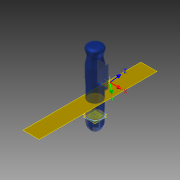
# Autodesk Inventor part: Handle_2
Saved by Autodesk Inventor 2011 SP2 (Build 150309200, 309)
## iProperties
Created: 2012-02-26
Part Number: Handle_2
Document SubType Name: Modeling
Designer: sungwook
Density: 1 g/cm^3
Author: sungwook
Autodesk Inventor part; units mm, degrees
note: some values were not read from the file. Chosen so that the rebuilt part matches the saved one: direction of "Hole2".
(part 1 of 20)
ref_plane "YZ Plane" through (0, 0, 0) normal (1, 0, 0) x (0, 1, 0)
sketch "Handle_0" plane through (0, 0, 0) normal (0, 0, 1) x (1, 0, 0)
  spline S0 degree 3 poles (-10017.42764, -10030.297385) (-10017.013951, -10030.15636) (-10016.17375, -10029.86994) (-10014.867675, -10029.493529) (-10013.491481, -10029.172596) (-10012.078899, -10028.93448) (-10010.677748, -10028.78461) (-10009.329448, -10028.709162) (-10008.026956, -10028.683902) (-10007.172289, -10028.683862) (-10006.749998, -10028.683842) knots 0 0 0 0 0.13110718 0.26627767 0.40758133 0.55482273 0.69573025 0.83010398 0.95981582 1.08650249 1.08650249 1.08650249 1.08650249
  spline S1 degree 3 poles (-10021.732129, -10032.297385) (-10021.73234, -10032.297385) (-10021.733186, -10032.297385) (-10021.73509, -10032.297385) (-10021.738258, -10032.297385) (-10021.742688, -10032.297385) (-10021.748373, -10032.297385) (-10021.755307, -10032.297385) (-10021.763486, -10032.297385) (-10021.772904, -10032.297385) (-10021.783555, -10032.297385) (-10021.795433, -10032.297385) (-10021.808523, -10032.297385) (-10021.822807, -10032.297385) (-10021.838268, -10032.297385) (-10021.854892, -10032.297385) (-10021.872666, -10032.297385) (-10021.884898, -10032.297385) (-10021.891203, -10032.297385) knots 0 0 0 0 0.00398745 0.01595749 0.03589091 0.06374884 0.09949715 0.14310174 0.1945285 0.2537433 0.32071204 0.39540061 0.47774624 0.56757484 0.66479437 0.76932497 0.8810868 1 1 1 1
  spline S2 degree 3 poles (-10021.891203, -10032.297385) (-10021.507581, -10032.143895) (-10020.74627, -10031.83929) (-10019.261429, -10031.164287) (-10018.160679, -10030.64392) (-10017.42764, -10030.297385) knots 0 0 0 0 0.25334256 0.50276707 1 1 1 1
  spline S3 degree 3 poles (-10017.79088, -10013.983385) (-10017.364369, -10014.133003) (-10016.497172, -10014.437213) (-10015.148667, -10014.843297) (-10013.724339, -10015.192835) (-10012.260529, -10015.454201) (-10010.808862, -10015.619234) (-10009.414249, -10015.702378) (-10008.068673, -10015.730197) (-10007.18611, -10015.730238) (-10006.749998, -10015.730259) knots 0 0 0 0 0.13558682 0.27568002 0.42231514 0.57532331 0.7214304 0.86036495 0.99429907 1.12513191 1.12513191 1.12513191 1.12513191
  line L0 (-10022.303899, -10015.983385) -> (-10006.749998, -10015.983385)
  line L1 (-10006.749998, -10015.730259) -> (-10006.749998, -10015.983385)
  line L2 (-10006.749998, -10015.983385) -> (-10006.749998, -10017.983385)
  spline S4 degree 3 poles (-10006.749998, -10017.983385) (-10007.632309, -10017.983385) (-10008.976773, -10017.983385) (-10010.804987, -10017.983385) (-10012.253003, -10017.983385) (-10013.713888, -10017.983385) (-10015.138402, -10017.983385) (-10016.48847, -10017.983385) (-10017.363516, -10017.983385) (-10017.791183, -10017.983385) knots 0 0 0 0 0.26469338 0.4033392 0.54846434 0.69909791 0.84160494 0.97581833 1.10411856 1.10411856 1.10411856 1.10411856
  spline S5 degree 3 poles (-10017.791183, -10017.983385) (-10018.527422, -10017.630624) (-10019.634362, -10017.100245) (-10020.947309, -10016.51954) (-10021.715083, -10016.204989) (-10022.106855, -10016.057543) (-10022.303899, -10015.983385) knots 0 0 0 0 0.49596798 0.74569065 0.8720938 1 1 1 1
  spline S6 degree 3 poles (-10022.303899, -10015.983385) (-10022.278889, -10015.901813) (-10022.229009, -10015.739129) (-10022.178389, -10015.489096) (-10022.146804, -10015.236972) (-10022.136391, -10014.983317) (-10022.146773, -10014.729742) (-10022.178339, -10014.477516) (-10022.22892, -10014.227552) (-10022.278782, -10014.064856) (-10022.303752, -10013.983385) knots 0 0 0 0 0.12572609 0.25074567 0.37552827 0.50000542 0.62458391 0.74924522 0.87443269 1 1 1 1
  spline S7 degree 3 poles (-10022.303752, -10013.983385) (-10021.914411, -10013.983385) (-10021.148705, -10013.983385) (-10019.644415, -10013.983385) (-10018.529465, -10013.983385) (-10017.79088, -10013.983385) knots 0 0 0 0 0.25882001 0.5090148 1 1 1 1
  line L3 (-10033.249998, -10030.297385) -> (-10017.42764, -10030.297385)
  line L4 (-10033.249998, -10030.297385) -> (-10033.249998, -10028.297385)
  line L5 (-10033.249998, -10028.297385) -> (-10006.749998, -10028.297385)
  line L6 (-10033.249998, -10032.297385) -> (-10021.891203, -10032.297385)
  line L7 (-10033.249998, -10032.297385) -> (-10033.249998, -10030.297385)
  line L8 (-10033.249998, -10017.983385) -> (-10017.791183, -10017.983385)
  line L9 (-10033.249998, -10017.983385) -> (-10033.249998, -10015.983385)
  line L10 (-10033.249998, -10015.983385) -> (-10022.303899, -10015.983385)
  line L11 (-10033.249998, -10015.983385) -> (-10033.249998, -10013.983385)
  line L12 (-10033.249998, -10013.983385) -> (-10022.303752, -10013.983385)
  line L13 (-10033.249998, -10018.729385) -> (-10006.749998, -10018.729385)
  line L14 (-10033.249998, -10018.729385) -> (-10033.249998, -10017.983385)
  line L15 (-10033.249998, -10016.729385) -> (-10006.749998, -10016.729385)
  line L16 (-10033.249998, -10014.729385) -> (-10017.28307, -10014.729385)
  spline S8 degree 3 poles (-10006.749998, -10016.350628) (-10007.166577, -10016.350609) (-10008.009501, -10016.35057) (-10009.293989, -10016.325181) (-10010.623578, -10016.249325) (-10012.005692, -10016.098622) (-10013.399659, -10015.859202) (-10014.758004, -10015.536726) (-10016.046768, -10015.158729) (-10016.875274, -10014.871005) (-10017.28307, -10014.729385) knots 0 0 0 0 0.12497306 0.25287553 0.38537145 0.52436553 0.66974205 0.80937847 0.9429718 1.07246485 1.07246485 1.07246485 1.07246485
  spline S9 degree 3 poles (-10022.047249, -10014.729385) (-10022.04174, -10014.815541) (-10022.030727, -10014.987752) (-10022.041635, -10015.246826) (-10022.072516, -10015.50434) (-10022.12485, -10015.759276) (-10022.197222, -10016.010445) (-10022.289119, -10016.256609) (-10022.398025, -10016.497644) (-10022.48411, -10016.651957) (-10022.527304, -10016.729385) knots 0 0 0 0 0.12386032 0.2475762 0.37158497 0.495852 0.6207493 0.74643209 0.87276965 1 1 1 1
  spline S10 degree 3 poles (-10022.527304, -10016.729385) (-10022.341346, -10016.801452) (-10021.971207, -10016.944898) (-10021.245451, -10017.252698) (-10020.356992, -10017.662141) (-10019.309622, -10018.185828) (-10018.619278, -10018.548029) (-10018.273621, -10018.729385) knots 0 0 0 0 0.12719878 0.25318248 0.50275428 0.75102731 1 1 1 1
  line L17 (-10035.749998, -10008.803385) -> (-10035.749998, -10032.803385)
  line L18 (-10149.710906, -10011.319385) -> (-10149.710906, -10030.287385)
  line L19 (-10149.325539, -10010.832703) -> (-10149.325539, -10030.774067)
  spline S11 degree 3 poles (-10130.726906, -10031.787385) (-10130.926034, -10031.641629) (-10131.327631, -10031.347673) (-10132.100995, -10030.700181) (-10132.860268, -10030.021094) (-10133.656819, -10029.374911) (-10134.185656, -10029.005591) (-10134.632315, -10028.744292) (-10134.982155, -10028.568235) (-10135.346656, -10028.411869) (-10135.59944, -10028.329114) (-10135.726906, -10028.287385) knots 0 0 0 0 0.07401284 0.14926686 0.30244691 0.37959616 0.45685507 0.49566205 0.53474567 0.5742877 0.61450742 0.61450742 0.61450742 0.61450742
  spline S12 degree 3 poles (-10130.726906, -10009.819385) (-10130.926034, -10009.965141) (-10131.327631, -10010.259097) (-10132.100995, -10010.906589) (-10132.860268, -10011.585676) (-10133.656819, -10012.231858) (-10134.185656, -10012.601179) (-10134.632315, -10012.862478) (-10134.982155, -10013.038535) (-10135.346656, -10013.194901) (-10135.59944, -10013.277656) (-10135.726906, -10013.319385) knots 0 0 0 0 0.07401284 0.14926686 0.30244691 0.37959616 0.45685507 0.49566205 0.53474567 0.5742877 0.61450742 0.61450742 0.61450742 0.61450742
  spline S13 degree 3 poles (-10125.726906, -10033.303385) (-10125.949716, -10033.300239) (-10126.395062, -10033.29395) (-10127.059625, -10033.234489) (-10127.71554, -10033.128934) (-10128.357478, -10032.969394) (-10128.981847, -10032.754825) (-10129.585717, -10032.484089) (-10130.170679, -10032.163086) (-10130.540701, -10031.913156) (-10130.726906, -10031.787385) knots 0 0 0 0 0.06683217 0.13358148 0.19996019 0.26595386 0.33177154 0.39774949 0.46426825 0.53165054 0.53165054 0.53165054 0.53165054
  spline S14 degree 3 poles (-10125.726906, -10008.303385) (-10125.949716, -10008.306531) (-10126.395062, -10008.312819) (-10127.059625, -10008.37228) (-10127.71554, -10008.477836) (-10128.357478, -10008.637376) (-10128.981847, -10008.851945) (-10129.585717, -10009.12268) (-10130.170679, -10009.443684) (-10130.540701, -10009.693614) (-10130.726906, -10009.819385) knots 0 0 0 0 0.06683217 0.13358148 0.19996019 0.26595386 0.33177154 0.39774949 0.46426825 0.53165054 0.53165054 0.53165054 0.53165054
  arc A0 (-10149.325539, -10010.832703) -> (-10149.710906, -10011.319385) centre (-10149.210906, -10011.319385) ccw
  arc A1 (-10149.710906, -10030.287385) -> (-10149.325539, -10030.774067) centre (-10149.210906, -10030.287385) ccw
  spline S15 degree 3 poles (-10135.726906, -10028.287385) (-10135.927757, -10028.233252) (-10136.338929, -10028.122433) (-10136.990756, -10028.038079) (-10137.683253, -10028.010641) (-10138.418457, -10028.048208) (-10139.194997, -10028.144543) (-10140.011682, -10028.296223) (-10140.865557, -10028.499181) (-10142.071793, -10028.832792) (-10143.629971, -10029.328885) (-10145.526237, -10029.953098) (-10147.128782, -10030.412477) (-10148.397883, -10030.680686) (-10149.021234, -10030.743434) (-10149.325539, -10030.774067) knots 0 0 0 0 0.06234657 0.1276327 0.1966407 0.27004939 0.34820305 0.43123424 0.51911498 0.61142292 0.80662861 1.00959387 1.21035176 1.30648489 1.39817641 1.39817641 1.39817641 1.39817641
  spline S16 degree 3 poles (-10135.726906, -10013.319385) (-10135.927757, -10013.373518) (-10136.338929, -10013.484337) (-10136.990756, -10013.56869) (-10137.683253, -10013.596129) (-10138.418457, -10013.558561) (-10139.194997, -10013.462227) (-10140.011682, -10013.310547) (-10140.865557, -10013.107589) (-10142.071793, -10012.773978) (-10143.629971, -10012.277884) (-10145.526237, -10011.653672) (-10147.128782, -10011.194293) (-10148.397883, -10010.926084) (-10149.021234, -10010.863335) (-10149.325539, -10010.832703) knots 0 0 0 0 0.06234657 0.1276327 0.1966407 0.27004939 0.34820305 0.43123424 0.51911498 0.61142292 0.80662861 1.00959387 1.21035176 1.30648489 1.39817641 1.39817641 1.39817641 1.39817641
  line L20 (-10150.726906, -10009.803385) -> (-10150.726906, -10031.803385)
  spline S17 degree 3 poles (-10135.726906, -10029.303385) (-10135.510838, -10029.403925) (-10135.07407, -10029.607162) (-10134.444184, -10029.982096) (-10133.812917, -10030.390211) (-10133.179963, -10030.831085) (-10132.5504, -10031.300817) (-10131.733284, -10031.962031) (-10131.128514, -10032.467631) (-10130.726906, -10032.803385) knots 0 0 0 0 0.07145122 0.1444341 0.21963753 0.29697342 0.37578786 0.45523025 0.61227239 0.61227239 0.61227239 0.61227239
  spline S18 degree 3 poles (-10135.726906, -10012.303385) (-10135.510838, -10012.202844) (-10135.07407, -10011.999608) (-10134.444184, -10011.624673) (-10133.812917, -10011.216558) (-10133.179963, -10010.775684) (-10132.5504, -10010.305952) (-10131.733284, -10009.644738) (-10131.128514, -10009.139138) (-10130.726906, -10008.803385) knots 0 0 0 0 0.07145122 0.1444341 0.21963753 0.29697342 0.37578786 0.45523025 0.61227239 0.61227239 0.61227239 0.61227239
  spline S19 degree 3 poles (-10130.726906, -10032.803385) (-10130.542266, -10032.946932) (-10130.26739, -10033.160633) (-10129.883991, -10033.41627) (-10129.594046, -10033.590111) (-10129.298537, -10033.745569) (-10128.997284, -10033.882043) (-10128.689809, -10033.998389) (-10128.376285, -10034.094702) (-10128.057096, -10034.171953) (-10127.623115, -10034.250453) (-10127.069205, -10034.306035) (-10126.399156, -10034.322456) (-10125.950896, -10034.320408) (-10125.726906, -10034.319385) knots 0 0 0 0 0.07013118 0.1044054 0.13817293 0.17150982 0.2045203 0.23732848 0.27006639 0.30285264 0.33579 0.40230943 0.46959172 0.53678969 0.53678969 0.53678969 0.53678969
  spline S20 degree 3 poles (-10130.726906, -10008.803385) (-10130.542266, -10008.659838) (-10130.26739, -10008.446137) (-10129.883991, -10008.1905) (-10129.594046, -10008.016658) (-10129.298537, -10007.8612) (-10128.997284, -10007.724726) (-10128.689809, -10007.608381) (-10128.376285, -10007.512068) (-10128.057096, -10007.434817) (-10127.623115, -10007.356317) (-10127.069205, -10007.300734) (-10126.399156, -10007.284313) (-10125.950896, -10007.286361) (-10125.726906, -10007.287385) knots 0 0 0 0 0.07013118 0.1044054 0.13817293 0.17150982 0.2045203 0.23732848 0.27006639 0.30285264 0.33579 0.40230943 0.46959172 0.53678969 0.53678969 0.53678969 0.53678969
  spline S21 degree 3 poles (-10149.710906, -10031.803385) (-10149.393866, -10031.786541) (-10148.726546, -10031.751088) (-10147.704936, -10031.538316) (-10146.631338, -10031.258666) (-10145.169176, -10030.808016) (-10143.727736, -10030.315182) (-10142.319952, -10029.845409) (-10141.332901, -10029.532903) (-10140.407015, -10029.271291) (-10139.548892, -10029.069685) (-10138.760999, -10028.933507) (-10138.041773, -10028.869988) (-10137.387135, -10028.879867) (-10136.78985, -10028.958693) (-10136.238524, -10029.099047) (-10135.89584, -10029.235913) (-10135.726906, -10029.303385) knots 0 0 0 0 0.09512154 0.200216 0.31218274 0.42803367 0.65906444 0.76919754 0.87325746 0.96964043 1.05776849 1.13759246 1.20931346 1.27406394 1.33359113 1.38967504 1.44420495 1.44420495 1.44420495 1.44420495
  spline S22 degree 3 poles (-10149.710906, -10009.803385) (-10149.393866, -10009.820228) (-10148.726546, -10009.855681) (-10147.704936, -10010.068454) (-10146.631338, -10010.348104) (-10145.169176, -10010.798753) (-10143.727736, -10011.291588) (-10142.319952, -10011.761361) (-10141.332901, -10012.073866) (-10140.407015, -10012.335479) (-10139.548892, -10012.537084) (-10138.760999, -10012.673262) (-10138.041773, -10012.736781) (-10137.387135, -10012.726902) (-10136.78985, -10012.648077) (-10136.238524, -10012.507723) (-10135.89584, -10012.370856) (-10135.726906, -10012.303385) knots 0 0 0 0 0.09512154 0.200216 0.31218274 0.42803367 0.65906444 0.76919754 0.87325746 0.96964043 1.05776849 1.13759246 1.20931346 1.27406394 1.33359113 1.38967504 1.44420495 1.44420495 1.44420495 1.44420495
  line L21 (-10149.710906, -10031.803385) -> (-10150.726906, -10031.803385)
  line L22 (-10149.710906, -10009.803385) -> (-10150.726906, -10009.803385)
  line L23 (-10006.749998, -10012.803385) -> (-10006.749998, -10015.730259)
  line L24 (-10006.749998, -10017.983385) -> (-10006.749998, -10028.683842)
  spline S23 degree 3 poles (-10031.749998, -10033.819385) (-10030.897738, -10033.818592) (-10029.621577, -10033.817404) (-10027.925572, -10033.716598) (-10026.664002, -10033.578136) (-10025.412467, -10033.368047) (-10024.172666, -10033.081692) (-10022.943295, -10032.726456) (-10022.136893, -10032.440778) (-10021.732129, -10032.297385) knots 0 0 0 0 0.25561003 0.38274706 0.50949551 0.6361782 0.76322409 0.89103186 1.01983443 1.01983443 1.01983443 1.01983443
  spline S24 degree 3 poles (-10031.749998, -10007.787385) (-10030.679979, -10007.791929) (-10029.078257, -10007.798732) (-10026.952775, -10007.982232) (-10025.377562, -10008.240759) (-10023.821321, -10008.617729) (-10021.7597, -10009.259937) (-10019.249998, -10010.295385) (-10016.740296, -10011.330833) (-10014.678674, -10011.973041) (-10013.122433, -10012.350011) (-10011.547221, -10012.608537) (-10009.421738, -10012.792037) (-10007.820017, -10012.79884) (-10006.749998, -10012.803385) knots 0 0 0 0 0.32084871 0.48028147 0.63946219 0.79924314 0.96029185 1.28673686 1.61318187 1.77423059 1.93401153 2.09319225 2.25262502 2.57347372 2.57347372 2.57347372 2.57347372
  line L25 (-10035.749998, -10015.803385) -> (-10006.749998, -10015.803385)
  line L26 (-10035.749998, -10025.803385) -> (-10006.749998, -10025.803385)
  line L27 (-10035.749998, -10015.840385) -> (-10033.249998, -10015.840385)
  line L28 (-10035.749998, -10017.618385) -> (-10033.249998, -10017.618385)
  line L29 (-10035.749998, -10015.094385) -> (-10033.249998, -10015.094385)
  line L30 (-10035.749998, -10016.872385) -> (-10033.249998, -10016.872385)
  line L31 (-10035.749998, -10029.408385) -> (-10033.249998, -10029.408385)
  line L32 (-10035.749998, -10031.186385) -> (-10033.249998, -10031.186385)
  line L33 (-10035.749998, -10032.803385) -> (-10095.749998, -10032.803385)
  line L34 (-10035.749998, -10008.803385) -> (-10095.749998, -10008.803385)
  line L35 (-10031.749998, -10033.819385) -> (-10095.749998, -10033.819385)
  line L36 (-10031.749998, -10007.787385) -> (-10095.749998, -10007.787385)
  spline S25 degree 3 poles (-10095.749998, -10032.803385) (-10095.95879, -10032.803722) (-10096.375966, -10032.804397) (-10097.001263, -10032.842396) (-10097.622612, -10032.929299) (-10098.238452, -10033.053385) (-10098.854291, -10033.17747) (-10099.47564, -10033.264374) (-10100.100937, -10033.302373) (-10100.518113, -10033.303047) (-10100.726906, -10033.303385) knots 0 0 0 0 0.0626312 0.12513986 0.18776052 0.25067229 0.31358405 0.37620471 0.43871337 0.50134457 0.50134457 0.50134457 0.50134457
  spline S26 degree 3 poles (-10095.749998, -10008.803385) (-10095.95879, -10008.803047) (-10096.375966, -10008.802373) (-10097.001263, -10008.764374) (-10097.622612, -10008.67747) (-10098.238452, -10008.553385) (-10098.854291, -10008.429299) (-10099.47564, -10008.342396) (-10100.100937, -10008.304397) (-10100.518113, -10008.303722) (-10100.726906, -10008.303385) knots 0 0 0 0 0.0626312 0.12513986 0.18776052 0.25067229 0.31358405 0.37620471 0.43871337 0.50134457 0.50134457 0.50134457 0.50134457
  spline S27 degree 3 poles (-10100.726906, -10034.319385) (-10100.518113, -10034.319047) (-10100.100937, -10034.318373) (-10099.47564, -10034.280374) (-10098.854291, -10034.19347) (-10098.238452, -10034.069385) (-10097.622612, -10033.945299) (-10097.001263, -10033.858396) (-10096.375966, -10033.820397) (-10095.95879, -10033.819722) (-10095.749998, -10033.819385) knots 0 0 0 0 0.0626312 0.12513986 0.18776052 0.25067229 0.31358405 0.37620471 0.43871337 0.50134457 0.50134457 0.50134457 0.50134457
  spline S28 degree 3 poles (-10100.726906, -10007.287385) (-10100.518113, -10007.287722) (-10100.100937, -10007.288397) (-10099.47564, -10007.326396) (-10098.854291, -10007.413299) (-10098.238452, -10007.537385) (-10097.622612, -10007.66147) (-10097.001263, -10007.748374) (-10096.375966, -10007.786373) (-10095.95879, -10007.787047) (-10095.749998, -10007.787385) knots 0 0 0 0 0.0626312 0.12513986 0.18776052 0.25067229 0.31358405 0.37620471 0.43871337 0.50134457 0.50134457 0.50134457 0.50134457
  line L37 (-10100.726906, -10033.303385) -> (-10125.726906, -10033.303385)
  line L38 (-10100.726906, -10008.303385) -> (-10125.726906, -10008.303385)
  line L39 (-10100.726906, -10034.319385) -> (-10125.726906, -10034.319385)
  line L40 (-10100.726906, -10007.287385) -> (-10125.726906, -10007.287385)
  point P0 (-10079.452988, -10020.745658)
  point P1 (-10016.183402, -10029.88413)
  point P2 (-10014.884456, -10029.51017)
  point P3 (-10013.507906, -10029.191138)
  point P4 (-10012.056042, -10028.945998)
  point P5 (-10010.655141, -10028.794439)
  point P6 (-10009.313659, -10028.716612)
  point P7 (-10008.016858, -10028.687938)
  point P8 (-10021.732763, -10032.297385)
  point P9 (-10021.734667, -10032.297385)
  point P10 (-10021.737838, -10032.297385)
  point P11 (-10021.74227, -10032.297385)
  point P12 (-10021.747956, -10032.297385)
  point P13 (-10021.754893, -10032.297385)
  point P14 (-10021.763073, -10032.297385)
  point P15 (-10021.772493, -10032.297385)
  point P16 (-10021.783146, -10032.297385)
  point P17 (-10021.795027, -10032.297385)
  point P18 (-10021.808126, -10032.297385)
  point P19 (-10021.822415, -10032.297385)
  point P20 (-10021.83788, -10032.297385)
  point P21 (-10021.854508, -10032.297385)
  point P22 (-10021.872287, -10032.297385)
  point P23 (-10020.74409, -10031.828089)
  point P24 (-10019.630269, -10031.329732)
  point P25 (-10016.508183, -10014.422776)
  point P26 (-10015.166413, -10014.825597)
  point P27 (-10013.741761, -10015.172806)
  point P28 (-10012.235518, -10015.441842)
  point P29 (-10010.783993, -10015.608583)
  point P30 (-10009.397288, -10015.694207)
  point P31 (-10008.058318, -10015.725752)
  point P32 (-10009.396932, -10017.983385)
  point P33 (-10010.78339, -10017.983385)
  point P34 (-10012.234641, -10017.983385)
  point P35 (-10013.740977, -10017.983385)
  point P36 (-10015.166047, -10017.983385)
  point P37 (-10016.508181, -10017.983385)
  point P38 (-10020.006848, -10016.940072)
  point P39 (-10021.135911, -10016.444356)
  point P40 (-10021.713878, -10016.208709)
  point P41 (-10022.232911, -10015.737598)
  point P42 (-10022.181511, -10015.48845)
  point P43 (-10022.15031, -10015.236461)
  point P44 (-10022.139855, -10014.983386)
  point P45 (-10022.15029, -10014.730103)
  point P46 (-10022.181431, -10014.478356)
  point P47 (-10022.232876, -10014.228868)
  point P48 (-10021.13573, -10013.983385)
  point P49 (-10020.006633, -10013.983385)
  point P50 (-10007.999722, -10016.346511)
  point P51 (-10009.278422, -10016.317691)
  point P52 (-10010.601069, -10016.239464)
  point P53 (-10011.982637, -10016.087129)
  point P54 (-10013.415365, -10015.840708)
  point P55 (-10014.774417, -10015.520065)
  point P56 (-10016.056433, -10015.144363)
  point P57 (-10022.035296, -10014.987953)
  point P58 (-10022.044942, -10015.246316)
  point P59 (-10022.076039, -10015.503598)
  point P60 (-10022.128036, -10015.758034)
  point P61 (-10022.200229, -10016.008863)
  point P62 (-10022.291677, -10016.255082)
  point P63 (-10022.401063, -10016.495378)
  point P64 (-10021.970605, -10016.948504)
  point P65 (-10021.424676, -10017.178898)
  point P66 (-10020.357865, -10017.668609)
  point P67 (-10019.312352, -10018.188708)
  point P68 (-10131.319394, -10031.343823)
  point P69 (-10131.899942, -10030.86499)
  point P70 (-10133.059876, -10029.864507)
  point P71 (-10133.662216, -10029.382441)
  point P72 (-10134.298196, -10028.94378)
  point P73 (-10134.633455, -10028.748334)
  point P74 (-10134.982498, -10028.572487)
  point P75 (-10135.346582, -10028.418214)
  point P76 (-10131.319394, -10010.262947)
  point P77 (-10131.899942, -10010.74178)
  point P78 (-10133.059876, -10011.742263)
  point P79 (-10133.662216, -10012.224329)
  point P80 (-10134.298196, -10012.66299)
  point P81 (-10134.633455, -10012.858436)
  point P82 (-10134.982498, -10013.034282)
  point P83 (-10135.346582, -10013.188556)
  point P84 (-10126.39499, -10033.285578)
  point P85 (-10127.059872, -10033.22659)
  point P86 (-10127.714976, -10033.11958)
  point P87 (-10128.35533, -10032.960006)
  point P88 (-10128.977669, -10032.745784)
  point P89 (-10129.580179, -10032.476916)
  point P90 (-10130.162759, -10032.155863)
  point P91 (-10126.39499, -10008.321192)
  point P92 (-10127.059872, -10008.38018)
  point P93 (-10127.714976, -10008.487189)
  point P94 (-10128.35533, -10008.646764)
  point P95 (-10128.977669, -10008.860985)
  point P96 (-10129.580179, -10009.129853)
  point P97 (-10130.162759, -10009.450906)
  point P98 (-10136.3323, -10028.138364)
  point P99 (-10136.97903, -10028.049098)
  point P100 (-10137.668551, -10028.021335)
  point P101 (-10138.401822, -10028.055945)
  point P102 (-10139.177671, -10028.150056)
  point P103 (-10139.994367, -10028.299807)
  point P104 (-10140.849879, -10028.500809)
  point P105 (-10141.740078, -10028.744985)
  point P106 (-10143.604291, -10029.323981)
  point P107 (-10145.537298, -10029.942828)
  point P108 (-10147.47235, -10030.477569)
  point P109 (-10148.414988, -10030.666228)
  point P110 (-10136.3323, -10013.468406)
  point P111 (-10136.97903, -10013.557672)
  point P112 (-10137.668551, -10013.585435)
  point P113 (-10138.401822, -10013.550825)
  point P114 (-10139.177671, -10013.456713)
  point P115 (-10139.994367, -10013.306963)
  point P116 (-10140.849879, -10013.105961)
  point P117 (-10141.740078, -10012.861785)
  point P118 (-10143.604291, -10012.282788)
  point P119 (-10145.537298, -10011.663942)
  point P120 (-10147.47235, -10011.1292)
  point P121 (-10148.414988, -10010.940541)
  point P122 (-10135.084221, -10029.615609)
  point P123 (-10134.453021, -10029.981993)
  point P124 (-10133.821232, -10030.389911)
  point P125 (-10133.186445, -10030.831646)
  point P126 (-10132.555245, -10031.303619)
  point P127 (-10131.935302, -10031.800388)
  point P128 (-10135.084221, -10011.991161)
  point P129 (-10134.453021, -10011.624777)
  point P130 (-10133.821232, -10011.216858)
  point P131 (-10133.186445, -10010.775123)
  point P132 (-10132.555245, -10010.303151)
  point P133 (-10131.935302, -10009.806382)
  point P134 (-10130.166297, -10033.224759)
  point P135 (-10129.881113, -10033.41487)
  point P136 (-10129.591256, -10033.588097)
  point P137 (-10129.296125, -10033.743121)
  point P138 (-10128.995318, -10033.879079)
  point P139 (-10128.688463, -10033.99517)
  point P140 (-10128.375566, -10034.091467)
  point P141 (-10128.056933, -10034.168711)
  point P142 (-10127.732881, -10034.22768)
  point P143 (-10127.071357, -10034.297459)
  point P144 (-10126.398885, -10034.3192)
  point P145 (-10130.166297, -10008.38201)
  point P146 (-10129.881113, -10008.191899)
  point P147 (-10129.591256, -10008.018672)
  point P148 (-10129.296125, -10007.863649)
  point P149 (-10128.995318, -10007.727691)
  point P150 (-10128.688463, -10007.611599)
  point P151 (-10128.375566, -10007.515303)
  point P152 (-10128.056933, -10007.438059)
  point P153 (-10127.732881, -10007.37909)
  point P154 (-10127.071357, -10007.309311)
  point P155 (-10126.398885, -10007.287569)
  point P156 (-10148.762521, -10031.730056)
  point P157 (-10147.729848, -10031.534937)
  point P158 (-10146.645971, -10031.254108)
  point P159 (-10145.537467, -10030.917414)
  point P160 (-10143.345179, -10030.188444)
  point P161 (-10142.299833, -10029.841771)
  point P162 (-10141.306861, -10029.530561)
  point P163 (-10140.378624, -10029.271051)
  point P164 (-10139.520037, -10029.072346)
  point P165 (-10138.732771, -10028.940446)
  point P166 (-10138.018036, -10028.88091)
  point P167 (-10137.370647, -10028.893174)
  point P168 (-10136.780629, -10028.972086)
  point P169 (-10136.237537, -10029.112056)
  point P170 (-10148.762521, -10009.876714)
  point P171 (-10147.729848, -10010.071832)
  point P172 (-10146.645971, -10010.352662)
  point P173 (-10145.537467, -10010.689356)
  point P174 (-10143.345179, -10011.418325)
  point P175 (-10142.299833, -10011.764998)
  point P176 (-10141.306861, -10012.076208)
  point P177 (-10140.378624, -10012.335718)
  point P178 (-10139.520037, -10012.534423)
  point P179 (-10138.732771, -10012.666324)
  point P180 (-10138.018036, -10012.72586)
  point P181 (-10137.370647, -10012.713596)
  point P182 (-10136.780629, -10012.634683)
  point P183 (-10136.237537, -10012.494714)
  point P184 (-10029.194146, -10033.78376)
  point P185 (-10027.925158, -10033.705954)
  point P186 (-10026.665405, -10033.566173)
  point P187 (-10025.416185, -10033.355701)
  point P188 (-10024.178001, -10033.071156)
  point P189 (-10022.950419, -10032.715451)
  point P190 (-10028.542321, -10007.85949)
  point P191 (-10026.954422, -10008.002524)
  point P192 (-10025.383559, -10008.259892)
  point P193 (-10023.829969, -10008.633192)
  point P194 (-10022.29191, -10009.110731)
  point P195 (-10019.249998, -10010.295385)
  point P196 (-10016.208086, -10011.480039)
  point P197 (-10014.670027, -10011.957577)
  point P198 (-10013.116436, -10012.330878)
  point P199 (-10011.545573, -10012.588245)
  dimension "d16" = 25
  dimension "d17" = 17
  dimension "d18" = 10
  dimension "d19" = 24
  dimension "d20" = 5
  dimension "d22" = 1.016
  dimension "d23" = 1.016
  dimension "d25" = 2
  dimension "d26" = 15
  dimension "d27" = 0.762
  dimension "d28" = 13
  dimension "d91" = 11
  dimension "d92" = 2
sketch "Top" plane through (0, 0, 0) normal (0, 0, 1) x (1, 0, 0)
  line L0 (-10061.384521, -10012.562071) -> (-10061.389559, -10012.537537)
  ellipse E0 centre (-10061.407327, -10012.439052) end of major axis (-10061.567958, -10011.655344) minor radius 0.002388 (-10061.441791, -10012.282554) -> (-10061.389559, -10012.537537) ccw
  ellipse E1 centre (-10061.407327, -10012.439052) end of major axis (-10061.567958, -10011.655344) minor radius 0.002388 (-10061.567958, -10011.655344) -> (-10061.477509, -10012.10741) ccw
  line L1 (-10061.567283, -10011.655206) -> (-10061.567958, -10011.655344)
  ellipse E2 centre (-10061.407327, -10025.75493) end of major axis (-10061.567958, -10026.538638) minor radius 0.002388 (-10061.477785, -10026.087929) -> (-10061.567958, -10026.538638) ccw
  line L2 (-10061.20265, -10024.741932) -> (-10061.155113, -10024.509464)
  line L3 (-10061.567283, -10026.538776) -> (-10061.567958, -10026.538638)
  ellipse E3 centre (-10061.263642, -10012.971414) end of major axis (-10061.51915, -10012.213314) minor radius 0.00228 (-10061.2891, -10012.902989) -> (-10061.238059, -10013.054418) ccw
  ellipse E4 centre (-10061.263642, -10012.971414) end of major axis (-10061.51915, -10012.213314) minor radius 0.00228 (-10061.328884, -10012.784757) -> (-10061.291067, -10012.897149) ccw
  ellipse E5 centre (-10061.263642, -10012.971414) end of major axis (-10061.51915, -10012.213314) minor radius 0.00228 (-10061.51915, -10012.213314) -> (-10061.462872, -10012.384811) ccw
  line L4 (-10061.511038, -10012.21058) -> (-10061.51915, -10012.213314)
  line L5 (-10061.409541, -10014.769939) -> (-10066.315364, -10016.423383)
  ellipse E6 centre (-10060.350214, -10010.329057) end of major axis (-10060.161446, -10011.106467) minor radius 0.136933 (-10060.411145, -10010.623849) -> (-10060.405836, -10010.640872) ccw
  line L6 (-10060.338992, -10010.911596) -> (-10060.389299, -10010.72101)
  ellipse E7 centre (-10059.392792, -10010.09658) end of major axis (-10059.274812, -10010.582461) minor radius 0.085583 (-10059.449723, -10010.216958) -> (-10059.256434, -10010.363491) ccw
  ellipse E8 centre (-10061.434014, -10028.787489) end of major axis (-10061.413862, -10029.587235) minor radius 0.133925 (-10061.545763, -10029.13876) -> (-10061.413862, -10029.587235) ccw
  line L7 (-10061.56724, -10028.814575) -> (-10061.614706, -10027.241099)
  line L8 (-10061.614706, -10027.241099) -> (-10061.417332, -10027.236126)
  ellipse E9 centre (-10059.462863, -10028.737822) end of major axis (-10059.442712, -10029.537568) minor radius 0.133925 (-10059.595504, -10028.465803) -> (-10059.596089, -10028.764908) ccw
  line L9 (-10061.614706, -10027.241099) -> (-10062.008153, -10027.251012)
  line L10 (-10062.683065, -10027.268018) -> (-10063.648706, -10027.292349)
  ellipse E10 centre (-10075.133509, -10029.132674) end of major axis (-10075.080864, -10031.222011) minor radius 0.349879 (-10075.432006, -10029.986721) -> (-10075.402988, -10030.241495) ccw
  ellipse E11 centre (-10074.246492, -10029.110324) end of major axis (-10074.193847, -10031.199661) minor radius 0.349879 (-10074.544121, -10029.973038) -> (-10074.51733, -10030.20858) ccw
  ellipse E12 centre (-10074.246492, -10029.110324) end of major axis (-10074.208708, -10030.609848) minor radius 0.251109 (-10074.479048, -10028.316655) -> (-10074.150585, -10030.566078) ccw
  ellipse E13 centre (-10059.462863, -10028.737822) end of major axis (-10059.450269, -10029.237663) minor radius 0.083703 (-10059.543871, -10028.811536) -> (-10059.384127, -10028.986292) ccw
  ellipse E14 centre (-10061.487283, -10026.335655) end of major axis (-10061.544418, -10027.133612) minor radius 0.002347 (-10061.497783, -10026.449782) -> (-10061.544418, -10027.133612) ccw
  line L11 (-10061.497783, -10026.449782) -> (-10061.493607, -10026.391115)
  line L12 (-10061.476769, -10026.154539) -> (-10061.387127, -10024.895089)
  line L13 (-10061.387127, -10024.895089) -> (-10061.173521, -10024.910383)
  line L14 (-10061.531232, -10027.134556) -> (-10061.544418, -10027.133612)
  line L15 (-10061.387127, -10024.895089) -> (-10063.052132, -10024.77587)
  line L16 (-10061.822261, -10012.975681) -> (-10061.480096, -10012.907935)
  line L17 (-10060.998732, -10013.943875) -> (-10061.270145, -10012.470589)
  ellipse E15 centre (-10061.381185, -10012.403223) end of major axis (-10061.536562, -10011.618457) minor radius 0.096422 (-10061.270145, -10012.470589) -> (-10061.562922, -10011.76131) ccw
  line L18 (-10061.562922, -10011.76131) -> (-10061.553965, -10012.28311)
  line L19 (-10061.52882, -10011.616924) -> (-10061.536562, -10011.618457)
  line L20 (-10061.704305, -10010.461504) -> (-10061.600471, -10010.450631)
  line L21 (-10061.396574, -10010.967179) -> (-10061.493208, -10010.091535)
  ellipse E16 centre (-10061.470276, -10009.985049) end of major axis (-10061.553594, -10009.189399) minor radius 0.034185 (-10061.559875, -10009.224682) -> (-10061.493208, -10010.091535) ccw
  ellipse E17 centre (-10075.282058, -10011.431377) end of major axis (-10075.499727, -10009.352743) minor radius 0.089309 (-10075.517106, -10009.495059) -> (-10075.497023, -10009.996264) ccw
  ellipse E18 centre (-10074.38777, -10011.33773) end of major axis (-10074.605438, -10009.259096) minor radius 0.089309 (-10074.622833, -10009.404086) -> (-10074.622381, -10009.471498) ccw
  ellipse E19 centre (-10059.482969, -10009.776944) end of major axis (-10059.430895, -10010.274225) minor radius 0.021366 (-10059.457656, -10010.153408) -> (-10059.439953, -10010.250814) ccw
  ellipse E20 centre (-10059.482969, -10009.776944) end of major axis (-10059.535043, -10009.279663) minor radius 0.021366 (-10059.539208, -10009.319581) -> (-10059.522494, -10009.589102) ccw
  ellipse E21 centre (-10060.147124, -10022.397006) end of major axis (-10060.001206, -10021.690837) minor radius 0.431228 (-10060.197722, -10023.105252) -> (-10060.134659, -10023.088549) ccw
  line L22 (-10062.092466, -10026.793121) -> (-10061.532714, -10026.851737)
  ellipse E22 centre (-10061.470276, -10028.208933) end of major axis (-10061.386958, -10027.413284) minor radius 0.034185 (-10061.507817, -10028.2395) -> (-10061.560262, -10028.942319) ccw
  line L23 (-10061.507817, -10028.2395) -> (-10061.40361, -10027.226433)
  line L24 (-10061.516659, -10026.656555) -> (-10062.081937, -10026.59736)
  ellipse E23 centre (-10075.282058, -10026.762604) end of major axis (-10075.499727, -10028.841239) minor radius 0.089309 (-10075.497023, -10028.197718) -> (-10075.517106, -10028.698922) ccw
  ellipse E24 centre (-10074.38777, -10026.856252) end of major axis (-10074.605438, -10028.934886) minor radius 0.089309 (-10074.622381, -10028.722483) -> (-10074.622833, -10028.789895) ccw
  ellipse E25 centre (-10074.38777, -10026.856252) end of major axis (-10074.543991, -10028.348094) minor radius 0.064098 (-10074.554367, -10028.307855) -> (-10074.525604, -10028.311215) ccw
  ellipse E26 centre (-10059.482969, -10028.417038) end of major axis (-10059.430895, -10027.919757) minor radius 0.021366 (-10059.426766, -10027.950635) -> (-10059.457656, -10028.040574) ccw
  ellipse E27 centre (-10059.482969, -10028.417038) end of major axis (-10059.535043, -10028.914319) minor radius 0.021366 (-10059.522494, -10028.60488) -> (-10059.52418, -10028.883049) ccw
  line L25 (-10064.124866, -10023.921474) -> (-10061.095983, -10024.521171)
  line L26 (-10061.548786, -10026.225478) -> (-10061.55557, -10026.303406)
  ellipse E28 centre (-10061.381185, -10025.790759) end of major axis (-10061.536562, -10026.575525) minor radius 0.096422 (-10061.55557, -10026.303406) -> (-10061.308549, -10025.915759) ccw
  line L27 (-10061.308549, -10025.915759) -> (-10060.980245, -10024.390161)
  line L28 (-10060.980245, -10024.390161) -> (-10060.933868, -10024.399344)
  line L29 (-10061.52882, -10026.577058) -> (-10061.536562, -10026.575525)
  line L30 (-10061.015543, -10024.445554) -> (-10060.980245, -10024.390161)
  line L31 (-10060.980245, -10024.390161) -> (-10064.107288, -10023.77103)
  line L32 (-10061.471703, -10012.107894) -> (-10061.483789, -10011.939815)
  ellipse E29 centre (-10061.487283, -10011.858327) end of major axis (-10061.544418, -10011.06037) minor radius 0.002347 (-10061.544418, -10011.06037) -> (-10061.483789, -10011.939815) ccw
  line L33 (-10061.531232, -10011.059425) -> (-10061.544418, -10011.06037)
  line L34 (-10064.180359, -10013.703572) -> (-10064.191247, -10013.704351)
  line L35 (-10061.773929, -10009.829957) -> (-10061.581428, -10009.834808)
  line L36 (-10061.571072, -10011.04786) -> (-10061.569401, -10009.517133)
  ellipse E30 centre (-10061.434014, -10009.406493) end of major axis (-10061.413862, -10008.606747) minor radius 0.133925 (-10061.413862, -10008.606747) -> (-10061.569401, -10009.517133) ccw
  ellipse E31 centre (-10075.133509, -10009.061308) end of major axis (-10075.186154, -10011.150645) minor radius 0.349879 (-10075.402988, -10007.952487) -> (-10075.432006, -10008.207261) ccw
  ellipse E32 centre (-10074.246492, -10009.083658) end of major axis (-10074.299136, -10011.172995) minor radius 0.349879 (-10074.51733, -10007.985402) -> (-10074.544121, -10008.220944) ccw
  ellipse E33 centre (-10074.246492, -10009.083658) end of major axis (-10074.208708, -10007.584134) minor radius 0.251109 (-10074.138818, -10007.647962) -> (-10074.479048, -10009.877327) ccw
  ellipse E34 centre (-10060.448438, -10009.431326) end of major axis (-10060.46859, -10010.231072) minor radius 0.133925 (-10060.583826, -10009.541967) -> (-10060.583804, -10009.561987) ccw
  ellipse E35 centre (-10059.462863, -10009.45616) end of major axis (-10059.475458, -10009.956001) minor radius 0.083703 (-10059.384127, -10009.20769) -> (-10059.385926, -10009.184511) ccw
  ellipse E36 centre (-10059.462863, -10009.45616) end of major axis (-10059.450269, -10008.956318) minor radius 0.083703 (-10059.518536, -10009.131265) -> (-10059.543871, -10009.382446) ccw
  line L37 (-10060.381968, -10027.39585) -> (-10060.355389, -10027.281524)
  ellipse E37 centre (-10060.350214, -10027.864925) end of major axis (-10060.538981, -10028.642335) minor radius 0.136933 (-10060.405836, -10027.55311) -> (-10060.411626, -10027.571687) ccw
  ellipse E38 centre (-10059.392792, -10028.097402) end of major axis (-10059.274812, -10027.61152) minor radius 0.085583 (-10059.256434, -10027.830491) -> (-10059.449723, -10027.977024) ccw
  ellipse E39 centre (-10061.263642, -10025.222568) end of major axis (-10061.51915, -10025.980668) minor radius 0.00228 (-10061.463306, -10025.810475) -> (-10061.51915, -10025.980668) ccw
  line L38 (-10060.31258, -10024.003001) -> (-10059.852584, -10024.158037)
  line L39 (-10061.511038, -10025.983402) -> (-10061.51915, -10025.980668)
  line L40 (-10062.997623, -10023.098042) -> (-10066.658236, -10021.86428)
  line L41 (-10059.978335, -10023.918759) -> (-10059.852584, -10024.158037)
  line L42 (-10059.852584, -10024.158037) -> (-10059.860224, -10024.181396)
  line L43 (-10059.96134, -10024.481113) -> (-10059.852584, -10024.158037)
  line L44 (-10061.343293, -10012.742645) -> (-10061.377815, -10012.5868)
  ellipse E40 centre (-10061.392821, -10012.50712) end of major axis (-10061.565584, -10011.725997) minor radius 0.002568 (-10061.40621, -10012.458453) -> (-10061.377815, -10012.5868) ccw
  ellipse E41 centre (-10061.392821, -10012.50712) end of major axis (-10061.565584, -10011.725997) minor radius 0.002568 (-10061.431875, -10012.342165) -> (-10061.40688, -10012.455424) ccw
  ellipse E42 centre (-10061.392821, -10012.50712) end of major axis (-10061.565584, -10011.725997) minor radius 0.002568 (-10061.565584, -10011.725997) -> (-10061.475615, -10012.143297) ccw
  line L45 (-10061.563556, -10011.725548) -> (-10061.565584, -10011.725997)
  ellipse E43 centre (-10059.345926, -10009.777641) end of major axis (-10059.434309, -10008.982539) minor radius 0.263102 (-10059.144207, -10010.464079) -> (-10059.098227, -10010.317873) ccw
  ellipse E44 centre (-10059.345926, -10009.777641) end of major axis (-10059.434309, -10008.982539) minor radius 0.263102 (-10059.214027, -10009.21629) -> (-10059.309467, -10009.051766) ccw
  ellipse E45 centre (-10059.345926, -10028.41634) end of major axis (-10059.434309, -10029.211443) minor radius 0.263102 (-10059.595846, -10028.945624) -> (-10059.550469, -10029.096622) ccw
  ellipse E46 centre (-10059.345926, -10028.41634) end of major axis (-10059.434309, -10029.211443) minor radius 0.263102 (-10059.535287, -10029.126915) -> (-10059.530071, -10029.135866) ccw
  ellipse E47 centre (-10059.345926, -10028.41634) end of major axis (-10059.434309, -10029.211443) minor radius 0.263102 (-10059.382965, -10029.202459) -> (-10059.214027, -10028.977692) ccw
  ellipse E48 centre (-10059.345926, -10028.41634) end of major axis (-10059.257544, -10027.621237) minor radius 0.263102 (-10059.098227, -10027.876108) -> (-10059.144207, -10027.729902) ccw
  line L46 (-10060.60321, -10014.691357) -> (-10060.649406, -10014.572421)
  ellipse E49 centre (-10061.194651, -10013.161802) end of major axis (-10061.48409, -10012.415997) minor radius 0.002457 (-10061.244487, -10013.040088) -> (-10061.238091, -10013.05659) ccw
  ellipse E50 centre (-10061.194651, -10013.161802) end of major axis (-10061.48409, -10012.415997) minor radius 0.002457 (-10061.281018, -10012.945755) -> (-10061.262274, -10012.994171) ccw
  ellipse E51 centre (-10061.194651, -10013.161802) end of major axis (-10061.48409, -10012.415997) minor radius 0.002457 (-10061.48409, -10012.415997) -> (-10061.457451, -10012.487532) ccw
  line L47 (-10059.670958, -10014.32956) -> (-10060.60321, -10014.691357)
  ellipse E52 centre (-10059.330147, -10012.438209) end of major axis (-10059.040708, -10013.184014) minor radius 0.002457 (-10059.215803, -10012.73906) -> (-10059.21498, -10012.728711) ccw
  line L48 (-10059.040708, -10013.184014) -> (-10059.97296, -10013.545811)
  line L49 (-10061.4689, -10012.410102) -> (-10061.48409, -10012.415997)
  line L50 (-10060.60321, -10014.691357) -> (-10065.582281, -10016.623679)
  line L51 (-10059.970688, -10013.544929) -> (-10059.670958, -10014.32956)
  line L52 (-10059.670958, -10014.32956) -> (-10059.856284, -10014.679937)
  ellipse E53 centre (-10059.981496, -10014.352157) end of major axis (-10060.366198, -10015.22694) minor radius 0.25544 (-10060.292913, -10015.22388) -> (-10059.856284, -10014.679937) ccw
  line L53 (-10060.292913, -10015.22388) -> (-10064.160115, -10016.724698)
  ellipse E54 centre (-10060.262399, -10012.800006) end of major axis (-10059.97296, -10013.545811) minor radius 0.002457 (-10060.031345, -10013.399417) -> (-10059.97296, -10013.545811) ccw
  line L54 (-10059.670958, -10014.32956) -> (-10060.030407, -10013.404113)
  ellipse E55 centre (-10059.330147, -10012.438209) end of major axis (-10059.149248, -10012.904337) minor radius 0.001536 (-10059.215594, -10012.736646) -> (-10059.215161, -10012.731199) ccw
  ellipse E56 centre (-10060.305787, -10010.468324) end of major axis (-10060.084143, -10011.237007) minor radius 0.14613 (-10060.393632, -10010.678018) -> (-10060.307433, -10010.909938) ccw
  line L55 (-10060.324592, -10010.910839) -> (-10060.39293, -10010.685746)
  ellipse E57 centre (-10059.361099, -10010.19593) end of major axis (-10059.222572, -10010.676357) minor radius 0.091331 (-10059.44944, -10010.219204) -> (-10059.227286, -10010.355086) ccw
  ellipse E58 centre (-10059.361099, -10010.19593) end of major axis (-10059.139455, -10010.964613) minor radius 0.14613 (-10059.407624, -10010.523127) -> (-10059.144207, -10010.464079) ccw
  line L56 (-10059.139455, -10010.964613) -> (-10059.524741, -10011.075708)
  line L57 (-10062.350001, -10018.491351) -> (-10062.806719, -10018.519709)
  line L58 (-10059.92499, -10023.576572) -> (-10059.788919, -10023.499298)
  line L59 (-10059.788919, -10023.499298) -> (-10059.895809, -10023.022488)
  ellipse E59 centre (-10059.377353, -10021.744695) end of major axis (-10059.172257, -10022.517958) minor radius 0.142054 (-10059.172257, -10022.517958) -> (-10059.155812, -10022.100307) ccw
  line L60 (-10059.172257, -10022.517958) -> (-10059.832489, -10022.693074)
  line L61 (-10061.593785, -10028.297289) -> (-10061.767102, -10028.306051)
  line L62 (-10061.69138, -10027.549966) -> (-10061.630912, -10027.546909)
  ellipse E60 centre (-10061.420853, -10028.89902) end of major axis (-10061.380459, -10029.697999) minor radius 0.142983 (-10061.54092, -10029.1817) -> (-10061.380459, -10029.697999) ccw
  line L63 (-10061.563894, -10028.901424) -> (-10061.641717, -10027.32851)
  line L64 (-10061.641717, -10027.32851) -> (-10061.612115, -10027.327014)
  ellipse E61 centre (-10059.455566, -10028.799661) end of major axis (-10059.415172, -10029.59864) minor radius 0.142983 (-10059.57111, -10029.119451) -> (-10059.309467, -10029.142215) ccw
  ellipse E62 centre (-10059.455566, -10028.799661) end of major axis (-10059.415172, -10029.59864) minor radius 0.142983 (-10059.603506, -10028.528877) -> (-10059.598608, -10028.802065) ccw
  line L65 (-10059.415172, -10029.59864) -> (-10061.380459, -10029.697999)
  line L66 (-10061.641717, -10027.32851) -> (-10061.676779, -10027.330283)
  line L67 (-10062.699473, -10027.381987) -> (-10063.520471, -10027.423494)
  line L68 (-10061.582979, -10028.515688) -> (-10061.793565, -10028.526334)
  ellipse E63 centre (-10075.079596, -10029.589563) end of major axis (-10074.974067, -10031.676897) minor radius 0.373543 (-10075.402988, -10030.241495) -> (-10074.974067, -10031.676897) ccw
  ellipse E64 centre (-10074.195217, -10029.544851) end of major axis (-10074.089688, -10031.632185) minor radius 0.373543 (-10074.51733, -10030.20858) -> (-10073.882635, -10031.179544) ccw
  line L69 (-10074.974067, -10031.676897) -> (-10074.089688, -10031.632185)
  ellipse E65 centre (-10074.195217, -10029.544851) end of major axis (-10074.119478, -10031.042938) minor radius 0.268093 (-10074.41067, -10028.324644) -> (-10074.01033, -10030.887189) ccw
  ellipse E66 centre (-10059.455566, -10028.799661) end of major axis (-10059.43032, -10029.299023) minor radius 0.089364 (-10059.544237, -10028.815209) -> (-10059.363417, -10028.985245) ccw
  line L70 (-10061.512851, -10025.662014) -> (-10061.943003, -10025.639407)
  line L71 (-10063.079908, -10025.023645) -> (-10062.885605, -10025.033857)
  line L72 (-10061.872185, -10025.087119) -> (-10061.426778, -10025.110528)
  ellipse E67 centre (-10061.492555, -10026.420654) end of major axis (-10061.534542, -10027.219552) minor radius 0.002573 (-10061.499896, -10026.511611) -> (-10061.534542, -10027.219552) ccw
  line L73 (-10061.499896, -10026.511611) -> (-10061.418356, -10024.949143)
  line L74 (-10061.418356, -10024.949143) -> (-10061.391076, -10024.950577)
  ellipse E68 centre (-10059.495322, -10026.525622) end of major axis (-10059.537309, -10027.324519) minor radius 0.002573 (-10059.515377, -10026.862757) -> (-10059.510196, -10026.85336) ccw
  line L75 (-10059.537309, -10027.324519) -> (-10061.534542, -10027.219552)
  line L76 (-10061.418356, -10024.949143) -> (-10063.059739, -10024.862878)
  line L77 (-10061.523137, -10025.823301) -> (-10061.758489, -10025.810932)
  ellipse E69 centre (-10059.495322, -10026.525622) end of major axis (-10059.521564, -10027.024932) minor radius 0.001608 (-10059.514117, -10026.860514) -> (-10059.511461, -10026.855695) ccw
  line L78 (-10061.500171, -10013.901093) -> (-10064.103785, -10014.452938)
  ellipse E70 centre (-10061.350908, -10012.457832) end of major axis (-10061.641194, -10011.088258) minor radius 0.211294 (-10061.435487, -10013.005451) -> (-10061.428862, -10013.029334) ccw
  line L79 (-10061.799477, -10013.0826) -> (-10061.435487, -10013.005451)
  line L80 (-10060.912741, -10014.033272) -> (-10060.961848, -10013.936717)
  line L81 (-10061.435487, -10013.005451) -> (-10061.474414, -10012.928914)
  line L82 (-10060.912741, -10014.033272) -> (-10061.22031, -10012.493439)
  ellipse E71 centre (-10061.350908, -10012.457832) end of major axis (-10061.516786, -10011.675218) minor radius 0.120739 (-10061.22031, -10012.493439) -> (-10061.554541, -10011.836276) ccw
  line L83 (-10061.554541, -10011.836276) -> (-10061.553361, -10012.752455)
  line L84 (-10059.945679, -10013.8283) -> (-10060.912741, -10014.033272)
  ellipse E72 centre (-10059.416785, -10012.047888) end of major axis (-10059.250907, -10012.830502) minor radius 0.120739 (-10059.215803, -10012.73906) -> (-10059.515377, -10011.331224) ccw
  line L85 (-10061.508918, -10011.67355) -> (-10061.516786, -10011.675218)
  line L86 (-10060.912741, -10014.033272) -> (-10064.079218, -10014.704417)
  line L87 (-10059.945679, -10013.8283) -> (-10060.203356, -10014.150069)
  ellipse E73 centre (-10060.364656, -10013.832921) end of major axis (-10060.929979, -10014.626526) minor radius 0.319988 (-10060.809239, -10014.642703) -> (-10060.203356, -10014.150069) ccw
  line L88 (-10060.809239, -10014.642703) -> (-10067.070029, -10015.969698)
  line L89 (-10059.945679, -10013.8283) -> (-10060.253248, -10012.288467)
  line L90 (-10061.526302, -10011.420587) -> (-10062.087976, -10011.483931)
  line L91 (-10061.695833, -10010.546688) -> (-10061.603118, -10010.536232)
  line L92 (-10061.378178, -10010.966212) -> (-10061.477952, -10010.09714)
  ellipse E74 centre (-10061.469475, -10010.020915) end of major axis (-10061.55913, -10009.225955) minor radius 0.01704 (-10061.56071, -10009.23864) -> (-10061.477952, -10010.09714) ccw
  ellipse E75 centre (-10059.482525, -10009.79683) end of major axis (-10059.392871, -10010.591791) minor radius 0.01704 (-10059.57111, -10009.07453) -> (-10059.407624, -10010.523127) ccw
  line L93 (-10061.567037, -10011.685094) -> (-10062.074207, -10011.742292)